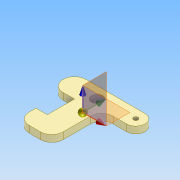
# Autodesk Inventor part: Selection_Lever 1
Saved by Autodesk Inventor 2018.1 (Build 221171000, 171)
## iProperties
Created: 2019-02-14
Part Number: Selection_Lever 1
Material: Nylon 6/6
Document SubType Name: Modeling
Designer: James
Density: 1.13 g/cm^3
Appearance: Nylon 6
Mass: 1.74334 g
Surface Area: 14.72 cm^2
Volume: 1.54278 cm^3
Author: James
Autodesk Inventor part; units mm, degrees
ref_plane "YZ Plane" through (0, 0, 0) normal (1, 0, 0) x (0, 1, 0)
ref_plane "XZ Plane" through (0, 0, 0) normal (0, 1, 0) x (-1, 0, 0)
ref_plane "XY Plane" through (0, 0, 0) normal (0, 0, 1) x (1, 0, 0)
sketch "Sketch1" plane through (0, 0, 0) normal (0, 0, 1) x (1, 0, 0)
  line L0 (0, 0) -> (20, 0)
  line L1 (20, 0) -> (20, 10)
  line L2 (20, 10) -> (0, 10)
  line L3 (0, 10) -> (0, 0)
  line L4 (20, 10) -> (35, 10)
  line L5 (35, 10) -> (35, 2)
  line L6 (35, 2) -> (20, 2)
  line L7 (20, 2) -> (20, 10)
  line L8 (20, 0) -> (10, 0)
  line L9 (10, 0) -> (10, -20)
  line L10 (10, -20) -> (20, -20)
  line L11 (20, -20) -> (20, 0)
  line L12 (10, -20) -> (5, -20)
  line L13 (5, -20) -> (5, -12)
  line L14 (5, -12) -> (10, -12)
  line L15 (10, -12) -> (10, -20)
  dimension "d0" = 10
  dimension "d1" = 20
  dimension "d2" = 15
  dimension "d3" = 8
  dimension "d4" = 20
  dimension "d5" = 8
  dimension "d6" = 5
  dimension "d7" = 10
  constraints: 32 end point, 8 parallel, 4 horizontal, 4 perpendicular
  measures "d0" distance of L2.end L0.start
  measures "d1" distance of L1.end L2.end
  measures "d2" distance of L1.end L4.end
  measures "d3" distance of L4.end L5.end
  measures "d4" distance between parallel lines of L0 L12
  measures "d5" distance of L12.end L13.end
  measures "d6" distance of L9.end L12.end
  measures "d7" distance of L9.end L10.end
extrude "Extrusion1" add sketch "Sketch1" along normal blind 3
fillet "Fillet1" radius 5 1 edges at (0, 10, 1.5)
fillet "Fillet2" radius 5 2 edges at (5, -20, 1.5) (20, -20, 1.5)
fillet "Fillet3" radius 5 1 edges at (20, 2, 1.5)
full round fillet "Fillet4" first side at (28.3333, 2, 1) centre faces at (35, 4.6667, 1) second side at (25, 10, 2)
sketch "Sketch2" plane through (0, 0, 3) normal (0, 0, 1) x (1, 0, 0)
  arc A0 (31, 2) -> (31, 10) centre (31, 6) ccw projected
  point P0 (0, 0)
  constraints: 1 coincident
hole "Hole1" at (31, 6, 3) direction (0, 0, -1) diameter 2 end through all
sketch "Sketch3" plane through (0, 0, 3) normal (0, 0, 1) x (1, 0, 0)
  line L0 (31, 10) -> (5, 10) projected
  line L1 (10, 0) -> (10, -12) projected
  point P0 (0, 0)
  point P1 (15, 5)
  dimension "d20" = 5
  dimension "d21" = 5
  measures "d20" distance from line of point (15, 5) L0
  measures "d21" distance from line of L1 point (15, 5)
hole "Hole2" at (15, 5, 3) direction (0, 0, -1) diameter 5 end through all
fillet "Fillet5" radius 5 1 edges at (0, 0, 1.5)
body "Solid1"
